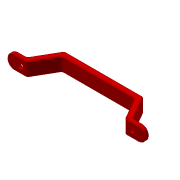
# Autodesk Inventor part: Door Handle
Saved by Autodesk Inventor 2015 (Build 190159000, 159)
## iProperties
Created: 2020-03-02
Part Number: Door Handle
Material: Generic
Document SubType Name: Modeling
Designer: Ghassan Yusuf
Density: 1 g/cm^3
Appearance: Default(1)
Author: Ghassan Yusuf
Autodesk Inventor part; units mm, degrees
ref_plane "YZ Plane" through (0, 0, 0) normal (1, 0, 0) x (0, 1, 0)
ref_plane "XZ Plane" through (0, 0, 0) normal (0, 1, 0) x (-1, 0, 0)
ref_plane "XY Plane" through (0, 0, 0) normal (0, 0, 1) x (1, 0, 0)
sketch "Sketch4" plane through (0, 0, 0) normal (0, 0, 1) x (1, 0, 0)
  line L0 (-37.5, 0) -> (-27.1077, 18)
  line L1 (-27.1077, 18) -> (27.1077, 18)
  line L2 (27.1077, 18) -> (37.5, 0)
  line L3 (-39.8094, 0) -> (-28.2624, 20)
  line L4 (-28.2624, 20) -> (28.2624, 20)
  line L5 (28.2624, 20) -> (39.8094, 0)
  line L6 (-35.1906, 0) -> (-25.953, 16)
  line L7 (-25.953, 16) -> (25.953, 16)
  line L8 (25.953, 16) -> (35.1906, 0)
  line L9 (-39.8094, 0) -> (-35.1906, 0)
  line L10 (35.1906, 0) -> (39.8094, 0)
  point P0 (0, 0)
  dimension "d13" = 120
  dimension "d14" = 120
  dimension "d17" = 75
  dimension "d18" = 18
  dimension "d23" = 37.5
  dimension "d25" = 2
  dimension "d63" = 2
  dimension "d64" = 70.3812
  constraints: 22 end point, 4 horizontal alignment, 3 horizontal, 2 other
  measures "d13" angle of L1 L0
  measures "d14" angle of L2 L1
  measures "d17" distance of L0.start L2.end
  measures "d18" distance from line of point (0, 0) L1
  measures "d23" distance of L0.start point (0, 0)
  measures "d25" distance between parallel lines of L0 L3
  measures "d63" distance between parallel lines of L0 L6
  measures "d64" distance of L8.end L6.start
extrude "Extrusion6" add sketch "Sketch4" along normal mid plane 10
sketch "Sketch9" plane through (-39.8094, 0, 5) normal (0, -1, 0) x (1, 0, 0)
  line L0 (-4.6188, -5) -> (4.6188, -5) construction
  line L1 (0, -10) -> (0, 0) projected
  line L2 (-4.6188, -10) -> (4.6188, -10)
  line L3 (4.6188, 0) -> (-4.6188, 0)
  arc A0 (-4.6188, 0) -> (-4.6188, -10) centre (-4.6188, -5) ccw
  line L4 (84.2376, -5) -> (75, -5) construction
  line L5 (68.0718, 0) -> (68.0718, -10) projected
  line L6 (79.6188, 0) -> (79.6188, -10) projected
  line L7 (84.2376, -10) -> (75, -10)
  line L8 (75, 0) -> (84.2376, 0)
  arc A1 (84.2376, -10) -> (84.2376, 0) centre (84.2376, -5) ccw
  line L9 (4.6188, 0) -> (4.6188, -10)
  line L10 (75, 0) -> (75, -10)
  line L11 (4.6188, 0) -> (4.6188, -10) projected
  line L12 (75, 0) -> (75, -10) projected
  point P0 (39.8094, -5)
  point P1 (0, -5)
  point P2 (79.6188, -5)
  constraints: 20 end point, 4 midpoint, 4 point on circle, 4 tangent, 3 collinear, 3 parallel, 3 point on line, 2 centre point, 1 coincident, 1 horizontal, 1 perpendicular, 1 vertical
extrude "Extrusion7" add sketch "Sketch9" against normal blind 3
sketch "Sketch10" plane through (-28.2624, 20, 5) normal (0, 1, 0) x (1, 0, 0)
  line L0 (0, 10) -> (56.5248, 10) construction
  line L1 (56.5248, 10) -> (56.5248, 0) construction
  line L2 (56.5248, 0) -> (0, 0) construction
  line L3 (0, 0) -> (0, 10) construction
  line L4 (0, 0) -> (0, 10) projected
  line L5 (56.5248, 0) -> (56.5248, 10) projected
  line L6 (0, 10) -> (56.5248, 10) projected
  line L7 (56.5248, 0) -> (0, 0) projected
  line L8 (3.0047, 1.95) -> (3.0047, 6.8883)
  line L9 (3.0047, 6.8883) -> (1.2004, 6.8883)
  line L10 (1.2004, 6.8883) -> (1.2004, 8.05)
  line L11 (1.2004, 8.05) -> (6.3414, 8.05)
  line L12 (6.3414, 8.05) -> (6.3414, 6.8883)
  line L13 (6.3414, 6.8883) -> (4.5372, 6.8883)
  line L14 (4.5372, 6.8883) -> (4.5372, 1.95)
  line L15 (4.5372, 1.95) -> (3.0047, 1.95)
  line L16 (6.3118, 1.95) -> (8.3731, 8.05)
  line L17 (8.3731, 8.05) -> (10.044, 8.05)
  line L18 (10.044, 8.05) -> (12.1053, 1.95)
  line L19 (12.1053, 1.95) -> (10.5284, 1.95)
  line L20 (10.5284, 1.95) -> (10.1478, 3.1957)
  line L21 (10.1478, 3.1957) -> (8.2298, 3.1957)
  line L22 (8.2298, 3.1957) -> (7.8442, 1.95)
  line L23 (7.8442, 1.95) -> (6.3118, 1.95)
  line L24 (9.8116, 4.303) -> (9.1888, 6.3199)
  line L25 (9.1888, 6.3199) -> (8.561, 4.303)
  line L26 (8.561, 4.303) -> (9.8116, 4.303)
  line L27 (18.057, 1.95) -> (16.2033, 1.95)
  line L28 (16.2033, 1.95) -> (14.5473, 4.4266)
  line L29 (14.5473, 4.4266) -> (14.2457, 4.0113)
  line L30 (14.2457, 4.0113) -> (14.2457, 1.95)
  line L31 (14.2457, 1.95) -> (12.7133, 1.95)
  line L32 (12.7133, 1.95) -> (12.7133, 8.05)
  line L33 (12.7133, 8.05) -> (14.2457, 8.05)
  line L34 (14.2457, 8.05) -> (14.2457, 5.3263)
  line L35 (14.2457, 5.3263) -> (16.2033, 8.05)
  line L36 (16.2033, 8.05) -> (17.968, 8.05)
  line L37 (17.968, 8.05) -> (15.793, 5.2175)
  line L38 (15.793, 5.2175) -> (18.057, 1.95)
  line L39 (18.5563, 1.95) -> (18.5563, 8.05)
  line L40 (18.5563, 8.05) -> (22.679, 8.05)
  line L41 (22.679, 8.05) -> (22.679, 6.8883)
  line L42 (22.679, 6.8883) -> (20.0788, 6.8883)
  line L43 (20.0788, 6.8883) -> (20.0788, 5.8156)
  line L44 (20.0788, 5.8156) -> (22.4763, 5.8156)
  line L45 (22.4763, 5.8156) -> (22.4763, 4.654)
  line L46 (22.4763, 4.654) -> (20.0788, 4.654)
  line L47 (20.0788, 4.654) -> (20.0788, 3.1117)
  line L48 (20.0788, 3.1117) -> (22.679, 3.1117)
  line L49 (22.679, 3.1117) -> (22.679, 1.95)
  line L50 (22.679, 1.95) -> (18.5563, 1.95)
  spline S0 degree 2 poles (29.2684, 5) (29.2684, 3.517) (27.6865, 1.8215) (26.3123, 1.8215) knots 0 0 0 1 2 2 2
  spline S1 degree 2 poles (26.3123, 1.8215) (24.9331, 1.8215) (23.3611, 3.5368) (23.3611, 5) knots 0 0 0 1 2 2 2
  spline S2 degree 2 poles (23.3611, 5) (23.3611, 6.4682) (24.9331, 8.1785) (26.3123, 8.1785) knots 0 0 0 1 2 2 2
  spline S3 degree 2 poles (26.3123, 8.1785) (27.6865, 8.1785) (29.2684, 6.478) (29.2684, 5) knots 0 0 0 1 2 2 2
  spline S4 degree 2 poles (27.6865, 5) (27.6865, 5.5487) (27.4641, 6.3149) (27.2713, 6.5571) knots 0 0 0 1 2 2 2
  spline S5 degree 2 poles (27.2713, 6.5571) (27.0785, 6.8092) (26.5842, 7.0267) (26.3172, 7.0267) knots 0 0 0 1 2 2 2
  spline S6 degree 2 poles (26.3172, 7.0267) (26.0355, 7.0267) (25.5757, 6.8241) (25.3632, 6.567) knots 0 0 0 1 2 2 2
  spline S7 degree 2 poles (25.3632, 6.567) (25.1753, 6.3297) (24.943, 5.5438) (24.943, 5) knots 0 0 0 1 2 2 2
  spline S8 degree 2 poles (24.943, 5) (24.943, 4.4365) (25.1654, 3.695) (25.3582, 3.4429) knots 0 0 0 1 2 2 2
  spline S9 degree 2 poles (25.3582, 3.4429) (25.551, 3.1908) (26.0503, 2.9733) (26.3172, 2.9733) knots 0 0 0 1 2 2 2
  spline S10 degree 2 poles (26.3172, 2.9733) (26.5891, 2.9733) (27.0933, 3.2056) (27.2762, 3.4528) knots 0 0 0 1 2 2 2
  spline S11 degree 2 poles (27.2762, 3.4528) (27.4739, 3.7197) (27.6865, 4.4266) (27.6865, 5) knots 0 0 0 1 2 2 2
  line L51 (35.403, 1.95) -> (33.9299, 1.95)
  line L52 (33.9299, 1.95) -> (31.5769, 6.2012)
  line L53 (31.5769, 6.2012) -> (31.5769, 1.95)
  line L54 (31.5769, 1.95) -> (30.1779, 1.95)
  line L55 (30.1779, 1.95) -> (30.1779, 8.05)
  line L56 (30.1779, 8.05) -> (32.0564, 8.05)
  line L57 (32.0564, 8.05) -> (34.004, 4.5551)
  line L58 (34.004, 4.5551) -> (34.004, 8.05)
  line L59 (34.004, 8.05) -> (35.403, 8.05)
  line L60 (35.403, 8.05) -> (35.403, 1.95)
  line L61 (36.6437, 1.95) -> (36.6437, 8.05)
  line L62 (36.6437, 8.05) -> (40.7664, 8.05)
  line L63 (40.7664, 8.05) -> (40.7664, 6.8883)
  line L64 (40.7664, 6.8883) -> (38.1662, 6.8883)
  line L65 (38.1662, 6.8883) -> (38.1662, 5.8156)
  line L66 (38.1662, 5.8156) -> (40.5637, 5.8156)
  line L67 (40.5637, 5.8156) -> (40.5637, 4.654)
  line L68 (40.5637, 4.654) -> (38.1662, 4.654)
  line L69 (38.1662, 4.654) -> (38.1662, 3.1117)
  line L70 (38.1662, 3.1117) -> (40.7664, 3.1117)
  line L71 (40.7664, 3.1117) -> (40.7664, 1.95)
  line L72 (40.7664, 1.95) -> (36.6437, 1.95)
  spline S12 degree 2 poles (48.5768, 3.7988) (48.5768, 3.3489) (48.2456, 2.6124) (47.9243, 2.3553) knots 0 0 0 1 2 2 2
  spline S13 degree 2 poles (47.9243, 2.3553) (47.603, 2.0983) (46.728, 1.8215) (46.1002, 1.8215) knots 0 0 0 1 2 2 2
  spline S14 degree 2 poles (46.1002, 1.8215) (45.3884, 1.8215) (44.3701, 2.0588) (44.0487, 2.2071) knots 0 0 0 1 2 2 2
  line L73 (44.0487, 2.2071) -> (44.0487, 3.5318)
  line L74 (44.0487, 3.5318) -> (44.197, 3.5318)
  spline S15 degree 2 poles (44.197, 3.5318) (44.5332, 3.3193) (45.4378, 3.0029) (45.8135, 3.0029) knots 0 0 0 1 2 2 2
  spline S16 degree 2 poles (45.8135, 3.0029) (46.0359, 3.0029) (46.555, 3.082) (46.7329, 3.2105) knots 0 0 0 1 2 2 2
  spline S17 degree 2 poles (46.7329, 3.2105) (46.8714, 3.3143) (47.0394, 3.6159) (47.0394, 3.8878) knots 0 0 0 1 2 2 2
  spline S18 degree 2 poles (47.0394, 3.8878) (47.0394, 4.1596) (46.8021, 4.4513) (46.6044, 4.5205) knots 0 0 0 1 2 2 2
  spline S19 degree 2 poles (46.6044, 4.5205) (46.4067, 4.5897) (45.858, 4.6045) (45.6454, 4.6045) knots 0 0 0 1 2 2 2
  line L75 (45.6454, 4.6045) -> (45.3834, 4.6045)
  line L76 (45.3834, 4.6045) -> (45.3834, 5.6772)
  line L77 (45.3834, 5.6772) -> (45.6256, 5.6772)
  spline S20 degree 2 poles (45.6256, 5.6772) (45.9025, 5.6772) (46.3721, 5.7267) (46.5352, 5.8008) knots 0 0 0 1 2 2 2
  spline S21 degree 2 poles (46.5352, 5.8008) (46.6983, 5.8799) (46.8812, 6.1567) (46.8812, 6.394) knots 0 0 0 1 2 2 2
  spline S22 degree 2 poles (46.8812, 6.394) (46.8812, 6.5818) (46.7082, 6.8142) (46.5846, 6.8784) knots 0 0 0 1 2 2 2
  spline S23 degree 2 poles (46.5846, 6.8784) (46.4363, 6.9526) (46.0409, 7.002) (45.9025, 7.002) knots 0 0 0 1 2 2 2
  spline S24 degree 2 poles (45.9025, 7.002) (45.68, 7.002) (45.2104, 6.8982) (44.9929, 6.8142) knots 0 0 0 1 2 2 2
  spline S25 degree 2 poles (44.9929, 6.8142) (44.8199, 6.7499) (44.4442, 6.5423) (44.3552, 6.4879) knots 0 0 0 1 2 2 2
  line L78 (44.3552, 6.4879) -> (44.2267, 6.4879)
  line L79 (44.2267, 6.4879) -> (44.2267, 7.7929)
  spline S26 degree 2 poles (44.2267, 7.7929) (44.5431, 7.9264) (45.6108, 8.1785) (46.1694, 8.1785) knots 0 0 0 1 2 2 2
  spline S27 degree 2 poles (46.1694, 8.1785) (46.7132, 8.1785) (47.514, 7.9907) (47.7957, 7.8078) knots 0 0 0 1 2 2 2
  spline S28 degree 2 poles (47.7957, 7.8078) (48.1072, 7.615) (48.4186, 7.0218) (48.4186, 6.6511) knots 0 0 0 1 2 2 2
  spline S29 degree 2 poles (48.4186, 6.6511) (48.4186, 6.1271) (47.8155, 5.346) (47.3212, 5.2323) knots 0 0 0 1 2 2 2
  line L80 (47.3212, 5.2323) -> (47.3212, 5.173)
  spline S30 degree 2 poles (47.3212, 5.173) (47.5387, 5.1434) (47.9539, 4.9852) (48.1517, 4.8072) knots 0 0 0 1 2 2 2
  spline S31 degree 2 poles (48.1517, 4.8072) (48.3346, 4.649) (48.5768, 4.1448) (48.5768, 3.7988) knots 0 0 0 1 2 2 2
  spline S32 degree 2 poles (55.0475, 4.9951) (55.0475, 4.1399) (54.3011, 2.7953) (53.7326, 2.4344) knots 0 0 0 1 2 2 2
  spline S33 degree 2 poles (53.7326, 2.4344) (53.2581, 2.128) (52.1409, 1.95) (51.5131, 1.95) knots 0 0 0 1 2 2 2
  line L81 (51.5131, 1.95) -> (49.605, 1.95)
  line L82 (49.605, 1.95) -> (49.605, 8.05)
  line L83 (49.605, 8.05) -> (51.4933, 8.05)
  spline S34 degree 2 poles (51.4933, 8.05) (52.1359, 8.05) (53.2581, 7.8869) (53.7524, 7.5705) knots 0 0 0 1 2 2 2
  spline S35 degree 2 poles (53.7524, 7.5705) (54.3505, 7.1849) (55.0475, 5.8799) (55.0475, 4.9951) knots 0 0 0 1 2 2 2
  spline S36 degree 2 poles (53.4756, 5.0049) (53.4756, 5.608) (53.0603, 6.4682) (52.6352, 6.7104) knots 0 0 0 1 2 2 2
  spline S37 degree 2 poles (52.6352, 6.7104) (52.3238, 6.8784) (51.6416, 6.913) (51.1671, 6.913) knots 0 0 0 1 2 2 2
  line L84 (51.1671, 6.913) -> (51.1374, 6.913)
  line L85 (51.1374, 6.913) -> (51.1374, 3.0919)
  line L86 (51.1374, 3.0919) -> (51.1671, 3.0919)
  spline S38 degree 2 poles (51.1671, 3.0919) (51.6812, 3.0919) (52.388, 3.1265) (52.7094, 3.3292) knots 0 0 0 1 2 2 2
  spline S39 degree 2 poles (52.7094, 3.3292) (53.085, 3.5665) (53.4756, 4.4019) (53.4756, 5.0049) knots 0 0 0 1 2 2 2
  point P0 (28.2624, 5)
  constraints: 4 collinear, 2 other
emboss "Emboss1" sketch "Sketch10" operation cut depth 1 direction (0, -1, 0) contours L8 L9 L10 L11 L12 L13 L14 L15 | L16 L17 L18 L19 L20 L21 L22 L23 | L27 L28 L29 L30 L31 L32 L33 L34 L35 L36 L37 L38 | L39 L40 L41 L42 L43 L44 L45 L46 L47 L48 L49 L50 | S0 S1 S2 S3 | L51 L52 L53 L54 L55 L56 L57 L58 L59 L60 | L61 L62 L63 L64 L65 L66 L67 L68 L69 L70 L71 L72 | S12 S13 S14 L73 L74 S15 S16 S17 S18 S19 L75 L76 L77 S20 S21 S22 S23 S24 S25 L78 L79 S26 S27 S28 S29 L80 S30 S31 | S32 S33 L81 L82 L83 S34 S35
sketch "Sketch11" plane through (-39.8094, 3, 5) normal (0, 1, 0) x (1, 0, 0)
  line L0 (3.1003, 5) -> (1.4548, 2.15)
  line L1 (1.4548, 2.15) -> (-1.836, 2.15)
  line L2 (-1.836, 2.15) -> (-3.4815, 5)
  line L3 (-3.4815, 5) -> (-1.836, 7.85)
  line L4 (-1.836, 7.85) -> (1.4548, 7.85)
  line L5 (1.4548, 7.85) -> (3.1003, 5)
  arc A0 (-4.6188, 10) -> (-4.6188, 0) centre (-4.6188, 5) ccw projected
  line L6 (83.1003, 5) -> (81.4548, 2.15)
  line L7 (81.4548, 2.15) -> (78.164, 2.15)
  line L8 (78.164, 2.15) -> (76.5185, 5)
  line L9 (76.5185, 5) -> (78.164, 7.85)
  line L10 (78.164, 7.85) -> (81.4548, 7.85)
  line L11 (81.4548, 7.85) -> (83.1003, 5)
  line L12 (84.2376, 10) -> (77.8868, 10) projected
  line L13 (1.7321, 10) -> (-4.6188, 10) projected
  line L14 (65.7624, 10) -> (13.8564, 10) projected
  line L15 (39.8094, 10) -> (39.8094, 0)
  line L16 (13.8564, 0) -> (65.7624, 0) projected
  point P0 (39.8094, 5)
  point P1 (-0.1906, 5)
  point P2 (-9.6188, 5)
  point P3 (79.8094, 5)
  dimension "d71" = 5.7
  dimension "d72" = 5.7
  dimension "d73" = 80
  dimension "d74" = 40
  constraints: 26 end point, 2 midpoint, 2 parallel, 1 horizontal alignment, 1 point on circle, 26 other
  measures "d71" distance between parallel lines of L1 L4
  measures "d72" distance between parallel lines of L7 L10
  measures "d73" distance of point (79.809, 5) point (-0.191, 5)
  measures "d74" distance from line of L15 point (-0.191, 5)
extrude "Extrusion8" cut sketch "Sketch11" along normal blind 5 and the other way blind 1.5
sketch "Sketch12" plane through (-39.8094, 1.5, 5) normal (0, 1, 0) x (1, 0, 0)
  circle A0 centre (-0.1906, 5) radius 2
  circle A1 centre (79.8094, 5) radius 2
  point P0 (39.8094, 5)
  dimension "d79" = 4
  dimension "d80" = 4
  constraints: 2 centre point
  measures "d79" diameter of A0
  measures "d80" diameter of A1
extrude "Extrusion9" cut sketch "Sketch12" against normal blind 5
fillet "Fillet4" radius 2 10 edges at (-38.0774, 3, 3.6849) (-38.0774, 3, -3.6849) (-35.1906, 0, 0) (-25.953, 16, 0) (-28.2624, 20, 0) (28.2624, 20, 0) (25.953, 16, 0) (35.1906, 0, 0) (38.0774, 3, -3.6849) (38.0774, 3, 3.6849)
fillet "Fillet5" radius 0.6 40 edges at (-25.7983, 15.7321, 5) (0, 16, 5) (25.7983, 15.7321, 5) (30.5718, 8, 5) (35.3453, 0.2679, 5) (40.3868, 0, 5) (49.4282, 0, 0) (40.3868, 0, -5) (35.3453, 0.2679, -5) (30.5718, 8, -5) (25.7983, 15.7321, -5) (0, 16, -5) (-25.7983, 15.7321, -5) (-30.5718, 8, -5) (-35.3453, 0.2679, -5) (-40.3868, 0, -5) (-49.4282, 0, 0) (-40.3868, 0, 5) (-35.3453, 0.2679, 5) (-30.5718, 8, 5) (-38.2321, 3.2679, 5) (-41.8301, 3, 5) (-49.4282, 3, 0) (-41.8301, 3, -5) (-38.2321, 3.2679, -5) (-33.1699, 11.5, -5) (-28.1077, 19.7321, -5) (0, 20, -5) (28.1077, 19.7321, -5) (33.1699, 11.5, -5) (38.2321, 3.2679, -5) (41.8301, 3, -5) (49.4282, 3, 0) (41.8301, 3, 5) (38.2321, 3.2679, 5) (33.1699, 11.5, 5) (28.1077, 19.7321, 5) (0, 20, 5) (-28.1077, 19.7321, 5) (-33.1699, 11.5, 5)
equation "\"d14\" = d13"
equation "\"d23\" = 0.5 * d17"
equation "\"d72\" = d71"
equation "\"d74\" = 0.5 * d73"
body "Solid3"
